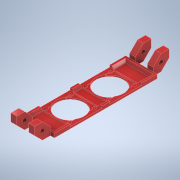
# Autodesk Inventor part: Prod05.3.3 - SKR1.4 Turbo Case Back 2
Saved by Autodesk Inventor 2021 (Build 250183000, 183)
## iProperties
Created: 2021-06-22
Part Number: Prod05.3.3 - SKR1.4 Turbo Case Back 2
Material: Generic
Document SubType Name: Modeling
Designer: alexr
Density: 1 g/cm^3
Appearance: Red
Author: alexr
Autodesk Inventor part; units mm, degrees
ref_plane "YZ Plane" through (0, 0, 0) normal (1, 0, 0) x (0, 1, 0)
ref_plane "XZ Plane" through (0, 0, 0) normal (0, 1, 0) x (-1, 0, 0)
ref_plane "XY Plane" through (0, 0, 0) normal (0, 0, 1) x (1, 0, 0)
sketch "Base Profile" plane through (0, 0, 0) normal (1, 0, 0) x (0, 1, 0)
  line L0 (10, 0) -> (20, 0)
  line L1 (20, 0) -> (20, -10)
  line L2 (10, -20) -> (5, -20)
  line L3 (0, -20) -> (0, -10)
  line L4 (0, -20) -> (0, -150)
  line L5 (5, -20) -> (5, -150)
  line L6 (5, -150) -> (10, -150)
  line L7 (20, -160) -> (20, -170)
  line L8 (20, -170) -> (10, -170)
  line L9 (0, -160) -> (0, -150)
  line L10 (0, -160) -> (10, -170)
  line L11 (10, 0) -> (0, -10)
  line L12 (20, -10) -> (10, -20)
  line L13 (10, -150) -> (20, -160)
  point P0 (0, 0)
  point P1 (20, -20)
  point P2 (10, -10)
  point P3 (20, -150)
  point P4 (0, -170)
  point P5 (10, -160)
  dimension "d0" = 20
  dimension "d1" = 20
  dimension "d3" = 130
  dimension "d4" = 5
  dimension "d5" = 20
  dimension "d6" = 20
  constraints: 28 end point, 8 point on line, 5 parallel, 2 horizontal, 2 perpendicular, 1 vertical
  measures "d0" distance of point (20, -20) L3.start
  measures "d1" distance of L0.end point (20, -20)
  measures "d3" distance of L3.start L4.end
  measures "d4" distance between parallel lines of L4 L5
  measures "d5" distance of L7.end point (0, -170)
  measures "d6" distance of point (20, -150) L7.end
extrude "Base Extrusion" add sketch "Base Profile" along normal blind 40
hole "Fixing Holes" at (0, 10, -160) at (0, 10, -10) direction (1, 0, 0) diameter 5.5 end through all
sketch "Cutouts and Structure" plane through (0, 5, -20) normal (0, 1, 0) x (1, 0, 0)
  line L0 (5, 5) -> (35, 5)
  line L1 (35, 125) -> (5, 125)
  line L2 (0, 130) -> (0, 0) projected
  line L3 (40, 130) -> (40, 0) projected
  line L4 (0, 0) -> (40, 0) projected
  line L5 (0, 130) -> (40, 130) projected
  line L6 (0, 20) -> (40, 20)
  line L7 (40, -10) -> (40, 140) projected
  line L8 (40, 60) -> (0, 60)
  line L9 (0, -10) -> (0, 140) projected
  line L10 (0, 70) -> (40, 70)
  line L11 (0, 110) -> (40, 110)
  line L12 (37, 127) -> (3, 127)
  line L13 (3, -10) -> (3, 0)
  line L14 (0, 65) -> (40, 65) construction
  line L15 (0, 21) -> (40, 21)
  line L16 (40, 59) -> (0, 59)
  line L17 (0, 71) -> (40, 71)
  line L18 (0, 109) -> (40, 109)
  arc A0 (5, 21.1716) -> (5, 26.8284) centre (4, 24) ccw
  arc A1 (5, 53.1716) -> (5, 58.8284) centre (4, 56) ccw
  line L19 (5, 53.1716) -> (5, 26.8284)
  line L20 (5, 21.1716) -> (5, 5)
  arc A2 (35, 26.8284) -> (35, 21.1716) centre (36, 24) ccw
  arc A3 (35, 58.8284) -> (35, 53.1716) centre (36, 56) ccw
  arc A4 (35, 76.8284) -> (35, 71.1716) centre (36, 74) ccw
  arc A5 (35, 108.8284) -> (35, 103.1716) centre (36, 106) ccw
  arc A6 (5, 103.1716) -> (5, 108.8284) centre (4, 106) ccw
  arc A7 (5, 71.1716) -> (5, 76.8284) centre (4, 74) ccw
  line L21 (5, 71.1716) -> (5, 58.8284)
  line L22 (5, 125) -> (5, 108.8284)
  line L23 (5, 103.1716) -> (5, 76.8284)
  line L24 (35, 108.8284) -> (35, 125)
  line L25 (35, 58.8284) -> (35, 71.1716)
  line L26 (35, 76.8284) -> (35, 103.1716)
  line L27 (35, 5) -> (35, 21.1716)
  line L28 (35, 26.8284) -> (35, 53.1716)
  line L29 (0, 130) -> (5.1, 130)
  line L30 (5.1, 130) -> (5.1, 150)
  line L31 (5.1, 150) -> (0, 150)
  line L32 (0, 150) -> (0, 130)
  line L33 (12.4, 130) -> (27.6, 130)
  line L34 (27.6, 130) -> (27.6, 150)
  line L35 (27.6, 150) -> (12.4, 150)
  line L36 (12.4, 150) -> (12.4, 130)
  line L37 (40, 140) -> (40, 150) projected
  line L38 (40, 150) -> (34.9, 150)
  line L39 (34.9, 150) -> (34.9, 130)
  line L40 (34.9, 130) -> (40, 130)
  line L41 (40, 130) -> (40, 150)
  line L42 (0, 0) -> (5.1, 0)
  line L43 (5.1, 0) -> (5.1, -20)
  line L44 (5.1, -20) -> (0, -20)
  line L45 (0, -20) -> (0, 0)
  line L46 (12.4, 0) -> (27.6, 0)
  line L47 (27.6, 0) -> (27.6, -20)
  line L48 (27.6, -20) -> (12.4, -20)
  line L49 (12.4, -20) -> (12.4, 0)
  line L50 (40, -20) -> (34.9, -20)
  line L51 (34.9, -20) -> (34.9, 0)
  line L52 (34.9, 0) -> (40, 0)
  line L53 (40, 0) -> (40, -20)
  point P0 (5, 109)
  point P1 (35, 109)
  point P2 (5, 71)
  point P3 (35, 71)
  point P4 (5, 59)
  point P5 (35, 59)
  point P6 (35, 21)
  point P7 (5, 21)
  point P8 (35, 20)
  point P9 (5, 20)
  point P10 (5, 110)
  point P11 (35, 110)
  point P12 (5, 70)
  point P13 (35, 70)
  point P14 (5, 60)
  point P15 (35, 60)
  point P16 (20, 40)
  point P17 (20, 90)
  dimension "d165" = 5
  dimension "d166" = 5
  dimension "d167" = 10
  dimension "d168" = 20
  dimension "d169" = 20
  dimension "d170" = 40
  dimension "d171" = 40
  dimension "d176" = 4
  dimension "d177" = 4
  dimension "d180" = 32
  dimension "d183" = 32
  dimension "d188" = 1
  dimension "d189" = 1
  dimension "d190" = 1
  dimension "d191" = 1
  dimension "d201" = 6
  dimension "d202" = 6
  dimension "d203" = 6
  dimension "d204" = 6
  dimension "d205" = 6
  dimension "d206" = 6
  dimension "d207" = 6
  dimension "d208" = 6
  dimension "d221" = 5.1
  dimension "d222" = 20
  dimension "d223" = 15.2
  dimension "d224" = 20
  dimension "d225" = 5.1
  dimension "d226" = 20
  dimension "d227" = 7.3
  constraints: 94 end point, 37 parallel, 16 point on circle, 15 symmetric about line, 10 perpendicular, 8 centre point, 8 coincident, 7 horizontal, 6 point on line, 1 midpoint, 1 vertical, 9 other
  measures "d165" distance between parallel lines of L4 L0
  measures "d166" distance between parallel lines of L5 L1
  measures "d167" distance between parallel lines of L10 L8
  measures "d168" distance between parallel lines of L4 L6
  measures "d169" distance between parallel lines of L5 L11
  measures "d170" distance between parallel lines of L8 L6
  measures "d171" distance between parallel lines of L11 L10
  measures "d176" distance from line of point (4, 24) L2
  measures "d177" distance from line of point (4, 24) L6
  measures "d180" distance of point (4, 24) point (4, 56)
  measures "d183" distance of point (4, 24) point (36, 24)
  measures "d188" distance between parallel lines of L6 L15
  measures "d189" distance between parallel lines of L8 L16
  measures "d190" distance between parallel lines of L10 L17
  measures "d191" distance between parallel lines of L11 L18
  measures "d201" diameter of A0
  measures "d202" diameter of A1
  measures "d203" diameter of A2
  measures "d204" diameter of A3
  measures "d205" diameter of A4
  measures "d206" diameter of A5
  measures "d207" diameter of A6
  measures "d208" diameter of A7
  measures "d221" distance of L31.end L30.end
  measures "d222" distance of L30.end L29.end
  measures "d223" distance of L35.end L34.end
  measures "d224" distance of L34.end L33.end
  measures "d225" distance of L40.end L39.end
  measures "d226" distance of L39.end L38.end
  measures "d227" distance between parallel lines of L34 L39
extrude "Structure Subtract" cut sketch "Cutouts and Structure" against normal blind 3.5 contours L20 L6 L27 L0 | L20 A0 L19 A1 L21 L16 L25 A3 L28 A2 L27 L15 | L21 L10 L25 L8 | L21 A7 L23 A6 L22 L18 L24 A5 L26 A4 L25 L17 | L22 L1 L24 L11
extrude "Fan Cutout Subtract" cut sketch "Cutouts and Structure" against normal blind 2.5 contours L20 L15 L27 L6 | L6 L2 L15 L20 | L27 L15 L3 L6 | L20 A0 L19 A1 L21 L16 L25 A3 L28 A2 L27 L15 | L15 L2 L16 L21 A1 L19 A0 L20 | L27 A2 L28 A3 L25 L16 L3 L15 | L2 L8 L21 L16 | L16 L25 L8 L3 | L21 L8 L25 L16 | L2 L17 L21 L10 | L10 L25 L17 L3 | L2 L18 L22 A6 L23 A7 L21 L17 | L21 L17 L25 L10 | L17 L25 A4 L26 A5 L24 L18 L3 | L2 L11 L22 L18 | L21 A7 L23 A6 L22 L18 L24 A5 L26 A4 L25 L17 | L18 L24 L11 L3 | L22 L11 L24 L18
hole "Fan Mounting Holes" at (4, 5, -44) at (4, 5, -76) at (36, 5, -44) at (36, 5, -76) at (4, 5, -126) at (4, 5, -94) at (36, 5, -94) at (36, 5, -126) direction (0, -1, 0) diameter 2.5 end through all
hole "Fan Airholes" at (20, 5, -60) at (20, 5, -110) direction (0, -1, 0) diameter 35 end through all
chamfer "Structure Clearance" distance 2.5 angle 45 8 edges at (35, 5, -137.5) (20, 5, -145) (5, 5, -137.5) (5, 5, -32.5) (20, 5, -25) (35, 5, -32.5) (5, 5, -85) (35, 5, -85)
extrude "Extrusion6" cut sketch "Cutouts and Structure" against normal through all both and the other way through all contours L4 L43 L44 L45 L9 | L7 L53 L50 L51 L4 | L47 L48 L49 L4 | L9 L32 L31 L30 L5 | L5 L39 L38 L37 L7 | L36 L35 L34 L5
equation "\"d168\" = d169"
body "Solid1"
